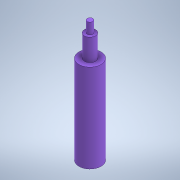
# Autodesk Inventor part: Marcador
Saved by Autodesk Inventor 2021 (Build 250183000, 183)
## iProperties
Created: 2022-10-27
Part Number: Marcador
Material: Generic
Document SubType Name: Modeling
Designer: USUARIO
Density: 1 g/cm^3
Appearance: Violet
Author: USUARIO
Autodesk Inventor part; units mm, degrees
ref_plane "YZ Plane" through (0, 0, 0) normal (1, 0, 0) x (0, 1, 0)
ref_plane "XZ Plane" through (0, 0, 0) normal (0, 1, 0) x (-1, 0, 0)
ref_plane "XY Plane" through (0, 0, 0) normal (0, 0, 1) x (1, 0, 0)
sketch "Sketch1" plane through (0, 0, 0) normal (0, 1, 0) x (-1, 0, 0)
  circle A0 centre (0, 0) radius 10
  circle A1 centre (0, 0) radius 5
  circle A2 centre (0, 0) radius 2.5
  dimension "d0" = 20
  dimension "d1" = 10
  dimension "d2" = 5
  constraints: 3 centre point, 3 coincident
  measures "d0" diameter of A0
  measures "d1" diameter of A1
  measures "d2" diameter of A2
extrude "Extrusion1" add sketch "Sketch1" along normal blind 80 contours A0
extrude "Extrusion2" add sketch "Sketch1" along normal blind 110 contours A2
extrude "Extrusion3" add sketch "Sketch1" along normal blind 100 contours A1
equation "\"d0\" = Dmarc"
equation "\"DER\" = 22"
equation "\"HR\" = 7"
equation "\"DIR\" = 8"
equation "\"DEM\" = 4"
equation "\"Dmarc\" = 20"
equation "\"Bsm\" = 22.5"
equation "\"Hsm\" = 12"
equation "\"Lsm\" = 21"
equation "\"Dsc\" = 5"
body "Solid1"
